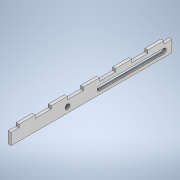
# Autodesk Inventor part: rail
Saved by Autodesk Inventor 2020 (Build 240168000, 168)
## iProperties
Created: 2019-12-21
Part Number: rail
Material: Générique
Document SubType Name: Modeling
Designer: damien
Density: 1 g/cm^3
Appearance: Par défaut
Author: damien
Autodesk Inventor part; units mm, degrees
ref_plane "YZ Plane" through (0, 0, 0) normal (1, 0, 0) x (0, 1, 0)
ref_plane "XZ Plane" through (0, 0, 0) normal (0, 1, 0) x (-1, 0, 0)
ref_plane "XY Plane" through (0, 0, 0) normal (0, 0, 1) x (1, 0, 0)
sketch "Esquisse1" plane through (0, 0, 0) normal (1, 0, 0) x (0, 1, 0)
  line L0 (0, 0) -> (-90, 0)
  line L1 (-90, 0) -> (-90, -1000)
  line L2 (-90, -1000) -> (0, -1000)
  line L3 (0, -1000) -> (0, 0)
  dimension "d0" = 1000
  dimension "d1" = 90
  constraints: 8 end point, 2 parallel, 1 horizontal, 1 perpendicular
  measures "d0" distance of L2.end L0.start
  measures "d1" distance of L0.start L0.end
extrude "Extrusion1" add sketch "Esquisse1" along normal blind 18.55
sketch "Esquisse2" plane through (18.55, 0, 0) normal (1, 0, 0) x (0, 0, -1)
  line L0 (150, 0) -> (250, 0)
  line L1 (250, 0) -> (250, -18.55)
  line L2 (250, -18.55) -> (150, -18.55)
  line L3 (150, -18.55) -> (150, 0)
  line L4 (0, 0) -> (0, -90) projected
  line L5 (1000, 0) -> (0, 0) projected
  line L6 (350, 0) -> (450, 0)
  line L7 (450, 0) -> (450, -18.55)
  line L8 (450, -18.55) -> (350, -18.55)
  line L9 (350, -18.55) -> (350, 0)
  line L10 (550, 0) -> (650, 0)
  line L11 (650, 0) -> (650, -18.55)
  line L12 (650, -18.55) -> (550, -18.55)
  line L13 (550, -18.55) -> (550, 0)
  line L14 (750, 0) -> (850, 0)
  line L15 (850, 0) -> (850, -18.55)
  line L16 (850, -18.55) -> (750, -18.55)
  line L17 (750, -18.55) -> (750, 0)
  line L18 (0, -18.55) -> (50, -18.55)
  line L19 (50, -18.55) -> (50, 0)
  line L20 (50, 0) -> (0, 0)
  line L21 (0, 0) -> (0, -18.55)
  line L22 (1000, 0) -> (950, 0)
  line L23 (950, 0) -> (950, -18.55)
  line L24 (950, -18.55) -> (1000, -18.55)
  line L25 (1000, -18.55) -> (1000, 0)
  point P0 (200, 0)
  point P1 (400, 0)
  point P2 (600, 0)
  point P3 (650, 0)
  point P4 (550, 0)
  point P5 (850, 0)
  point P6 (750, 0)
  point P7 (450, 0)
  point P8 (350, 0)
  point P9 (950, 0)
  dimension "d5" = 100
  dimension "d6" = 18.55
  dimension "d9" = 200
  dimension "d25" = 100
  dimension "d26" = 50
  dimension "d27" = 50
  dimension "d28" = 100
  constraints: 48 end point, 6 parallel, 4 horizontal, 3 collinear, 3 perpendicular, 2 point on line, 27 other
  measures "d5" distance of L0.start L0.end
  measures "d6" distance of L0.end L1.end
  measures "d9" distance of L4.start point (200, 0)
  measures "d25" distance between parallel lines of L3 L19
  measures "d26" distance of L23.end L24.end
  measures "d27" distance of L18.start L18.end
  measures "d28" distance between parallel lines of L23 L15
extrude "Extrusion2" cut sketch "Esquisse2" against normal blind 18.55
sketch "Esquisse3" plane through (18.55, 0, 0) normal (1, 0, 0) x (0, 0, -1)
  line L0 (550, -55) -> (950, -55) construction
  line L1 (550, -70) -> (950, -70)
  line L2 (950, -40) -> (550, -40)
  arc A0 (550, -40) -> (550, -70) centre (550, -55) ccw
  arc A1 (950, -70) -> (950, -40) centre (950, -55) ccw
  line L3 (1000, -90) -> (1000, 0) projected
  line L4 (0, -90) -> (1000, -90) projected
  circle A2 centre (350, -55) radius 15
  line L5 (0, 0) -> (0, -90) projected
  point P0 (750, -55)
  point P1 (700, -18.55)
  point P2 (0, -18.55)
  dimension "d16" = 15
  dimension "d17" = 50
  dimension "d18" = 400
  dimension "d19" = 35
  dimension "d20" = 350
  dimension "d21" = 30
  constraints: 8 end point, 4 point on circle, 4 tangent, 3 centre point, 1 horizontal, 1 midpoint, 1 parallel, 1 point on line, 1 other
  measures "d16" radius of A1
  measures "d18" distance of L0.start L0.end
  measures "d19" distance between parallel lines of L4 L0
  measures "d20" distance from line of L5 A2.centre
  measures "d21" diameter of A2
extrude "Extrusion3" cut sketch "Esquisse3" against normal blind 18.55
